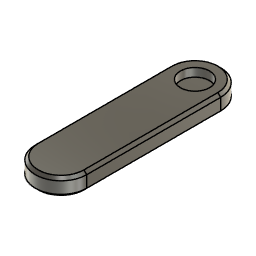
crank-arm (Autodesk Fusion 360 design; units mm, degrees)
Autodesk Fusion 360 part; units mm, degrees
sketch "main" plane through (0, 0, 0) normal (0, 0, 1) x (1, 0, 0) in component "crank-arm"
  circle A0 centre (0, 0) radius 13.05
  circle A1 centre (0, 0) radius 23
  line L0 (-23, 0) -> (23, 0)
  line L1 (23, 0) -> (23, -120)
  line L2 (23, -120) -> (-23, -120)
  line L3 (-23, -120) -> (-23, 0)
  circle A2 centre (0, -120) radius 23
  circle A3 centre (0, -120) radius 13.05
  dimension "d1" = 26.1
  dimension "d2" = 46
  dimension "d3" = 46
  dimension "d4" = 120
  dimension "d5" = 46
  dimension "d6" = 26.1
  constraint coincident A0.centre A1.centre
  constraint concentric A0 A1
  constraint horizontal L0
  constraint vertical L1
  constraint horizontal L2
  constraint vertical L3
  constraint coincident A1 L0.start
  constraint midpoint L2 A2.centre
  constraint concentric A2 A3
  measures "d1" diameter of A0
  measures "d2" diameter of A1
  measures "d3" distance of L0.start L0.end
  measures "d4" distance of L0.start L2.end
  measures "d5" diameter of A2
  measures "d6" diameter of A3
extrude "Extrude1" add sketch "main" along normal blind 8 contours A0 L0 | A0 A1 L0 | A0 A1 L0 | A0 L0 | A1 L1 L3 A2 | L2 A2 A3 | L2 A2 A3 in component "crank-arm"
extrude "Extrude2" add sketch "main" along normal blind 7.5 from surface at 8 contours A0 A1 L0 | A0 A1 L0 | A1 L1 L3 A2 | L2 A2 A3 | L2 A2 A3 | L2 A3 | L2 A3 in component "crank-arm"
chamfer "Chamfer1" distance 2.5 angle 45 8 edges at (-23, -60, 15.5) (0, -143, 15.5) (23, -60, 15.5) (0, 23, 15.5) (-23, -60, 0) (0, 23, 0) (23, -60, 0) (0, -143, 0) in component "crank-arm"
component "crank-arm" placed x (1, 0, 0) y (0, 1, 0) z (0, 0, 1) at (0, 0, 0)
equation "d1 = 26 mm + 0.1 mm"
equation "d6 = 26 mm + 0.1 mm"
equation "d10 = 8 mm - 0.5 mm"
named bodies: "crank-arm"
